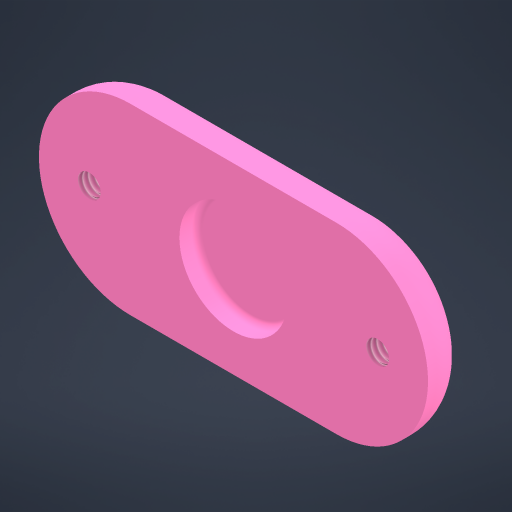
# Autodesk Inventor part: AxleCovers
Saved by Autodesk Inventor 2024.2 (Build 282272000, 272)
## iProperties
Created: 2023-09-28
Part Number: AxleCovers
Material: Generic
Document SubType Name: Modeling
Designer: tech
Density: 1 g/cm^3
Appearance: Machined - Aluminum
Author: tech
Autodesk Inventor part; units mm, degrees
ref_plane "YZ Plane" through (0, 0, 0) normal (1, 0, 0) x (0, 1, 0)
ref_plane "XZ Plane" through (0, 0, 0) normal (0, 1, 0) x (-1, 0, 0)
ref_plane "XY Plane" through (0, 0, 0) normal (0, 0, 1) x (1, 0, 0)
sketch "Sketch10" plane through (0, 0, 0) normal (0, 0, 1) x (1, 0, 0)
  circle A0 centre (0, 0) radius 6
  line L0 (0, 0) -> (16.002, 0)
  line L1 (0, 0) -> (-16.002, 0)
  circle A1 centre (-16.002, 0) radius 1.27
  circle A2 centre (16.002, 0) radius 1.27
  line L2 (-11.43, 10.16) -> (11.43, 10.16)
  line L3 (21.59, 0) -> (21.59, 0)
  line L4 (11.43, -10.16) -> (-11.43, -10.16)
  line L5 (-21.59, 0) -> (-21.59, 0)
  arc A3 (-11.43, 10.16) -> (-21.59, 0) centre (-11.43, 0) ccw
  arc A4 (-21.59, 0) -> (-11.43, -10.16) centre (-11.43, 0) ccw
  arc A5 (11.43, -10.16) -> (21.59, 0) centre (11.43, 0) ccw
  arc A6 (21.59, 0) -> (11.43, 10.16) centre (11.43, 0) ccw
  point P0 (0, -10.16)
  dimension "d40" = 12
  dimension "d41" = 16.002
  dimension "d42" = 16.002
  dimension "d43" = 2.54
  dimension "d44" = 2.54
  dimension "d45" = 10.16
  dimension "d46" = 10.16
  dimension "d47" = 21.59
  dimension "d48" = 21.59
  dimension "d49" = 10.16
  dimension "d50" = 10.16
  dimension "d51" = 10.16
  dimension "d52" = 10.16
  constraints: 12 end point, 8 point on circle, 8 tangent, 7 centre point, 3 coincident, 3 horizontal, 2 parallel, 1 midpoint, 1 perpendicular
  measures "d40" diameter of A0
  measures "d41" distance of L0.start L0.end
  measures "d42" distance of L0.start L1.end
  measures "d43" diameter of A1
  measures "d44" diameter of A2
  measures "d45" distance from line of L2 point (0, 0)
  measures "d46" distance of point (0, -10.16) point (0, 0)
  measures "d47" distance from line of point (0, 0) L3
  measures "d48" distance from line of L5 point (0, 0)
  measures "d49" radius of A3
  measures "d50" radius of A4
  measures "d51" radius of A5
  measures "d52" radius of A6
extrude "Extrusion11" add sketch "Sketch10" against normal blind 5 contours L0 L1 A0 | A1 | A0 L1 L0 | A2 | L2 A6 A5 L4 A4 A3
extrude "Extrusion12" cut sketch "Sketch10" against normal blind 2 contours L0 L1 A0 | A0 L1 L0
fillet "Fillet2" radius 0.635 1 edges at (-6, 0, -2)
fillet "Fillet3" radius 4 4 edges at (0, -10.16, -5) (-21.59, 0, -5) (0, 10.16, -5) (21.59, 0, -5)
extrude "Extrusion13" cut sketch "Sketch10" against normal blind 3.5 contours A1 | A2
thread "Thread1" size "4-40 UNC" class "2B" standard "ANSI Unified Screw Threads" full length
thread "Thread2" size "4-40 UNC" class "2B" standard "ANSI Unified Screw Threads" full length
sketch "Sketch11" plane through (0, 0, -5) normal (0, 0, -1) x (-1, 0, 0)
  line L0 (-21.5717, 10.2034) -> (21.5609, 10.2034) construction
  line L1 (21.5609, 10.2034) -> (21.5609, -10.088) construction
  line L2 (21.5609, -10.088) -> (-21.5717, -10.088) construction
  line L3 (-21.5717, -10.088) -> (-21.5717, 10.2034) construction
  spline S0 degree 2 poles (-8.7726, -2.4036) (-8.7726, -3.0619) (-9.24, -4.0827) (-10.1273, -4.7886) (-11.4247, -5.1511) (-12.2547, -5.1511) knots 0 0 0 1 2 3 4 4 4
  spline S1 degree 2 poles (-12.2547, -5.1511) (-13.0369, -5.1511) (-14.2676, -4.8268) (-15.1357, -4.1781) (-15.5841, -3.2431) (-15.5841, -2.6421) knots 0 0 0 1 2 3 4 4 4
  spline S2 degree 2 poles (-15.5841, -2.6421) (-15.5841, -2.1651) (-15.2693, -1.3638) (-14.6873, -0.696) (-13.8287, -0.1045) (-13.285, 0.1626) knots 0 0 0 1 2 3 4 4 4
  spline S3 degree 2 poles (-13.285, 0.1626) (-13.7524, 0.4011) (-14.4774, 0.9449) (-14.9735, 1.5745) (-15.2311, 2.29) (-15.2311, 2.7193) knots 0 0 0 1 2 3 4 4 4
  spline S4 degree 2 poles (-15.2311, 2.7193) (-15.2311, 3.244) (-14.8495, 4.1789) (-14.0768, 4.8658) (-12.8843, 5.2665) (-12.0829, 5.2665) knots 0 0 0 1 2 3 4 4 4
  spline S5 degree 2 poles (-12.0829, 5.2665) (-11.3197, 5.2665) (-10.2036, 4.8944) (-9.4785, 4.2648) (-9.1351, 3.4062) (-9.1351, 2.9101) knots 0 0 0 1 2 3 4 4 4
  spline S6 degree 2 poles (-9.1351, 2.9101) (-9.1351, 2.5094) (-9.3927, 1.7749) (-9.8888, 1.1261) (-10.6138, 0.5537) (-11.0908, 0.2962) knots 0 0 0 1 2 3 4 4 4
  spline S7 degree 2 poles (-11.0908, 0.2962) (-10.5279, 0.029) (-9.6598, -0.5529) (-9.0779, -1.2207) (-8.7726, -1.9648) (-8.7726, -2.4036) knots 0 0 0 1 2 3 4 4 4
  spline S8 degree 2 poles (-10.1368, -2.5467) (-10.1368, -2.1842) (-10.4039, -1.6023) (-10.9381, -1.0871) (-11.7395, -0.6101) (-12.2737, -0.3525) knots 0 0 0 1 2 3 4 4 4
  spline S9 degree 2 poles (-12.2737, -0.3525) (-12.7603, -0.6006) (-13.5044, -1.0871) (-13.9814, -1.6023) (-14.2199, -2.1747) (-14.2199, -2.5181) knots 0 0 0 1 2 3 4 4 4
  spline S10 degree 2 poles (-14.2199, -2.5181) (-14.2199, -3.2718) (-13.18, -4.1017) (-12.1593, -4.1017) knots 0 0 0 1 2 2 2
  spline S11 degree 2 poles (-12.1593, -4.1017) (-11.1576, -4.1017) (-10.1368, -3.2622) (-10.1368, -2.5467) knots 0 0 0 1 2 2 2
  spline S12 degree 2 poles (-10.4611, 2.7861) (-10.4611, 3.1104) (-10.6901, 3.6447) (-11.1289, 4.0263) (-11.7681, 4.2171) (-12.1879, 4.2171) knots 0 0 0 1 2 3 4 4 4
  spline S13 degree 2 poles (-12.1879, 4.2171) (-13.0274, 4.2171) (-13.8955, 3.4539) (-13.8955, 2.7861) knots 0 0 0 1 2 2 2
  spline S14 degree 2 poles (-13.8955, 2.7861) (-13.8955, 2.4808) (-13.6856, 1.9561) (-13.2373, 1.4887) (-12.5599, 1.0403) (-12.0925, 0.8018) knots 0 0 0 1 2 3 4 4 4
  spline S15 degree 2 poles (-12.0925, 0.8018) (-11.3007, 1.212) (-10.4611, 2.1946) (-10.4611, 2.7861) knots 0 0 0 1 2 2 2
  spline S16 degree 2 poles (-0.4633, -2.127) (-0.4633, -2.3845) (-0.6255, -2.6803) (-0.7591, -2.6803) knots 0 0 0 1 2 2 2
  line L4 (-0.7591, -2.6803) -> (-1.9039, -2.6803)
  line L5 (-1.9039, -2.6803) -> (-1.9039, -4.8077)
  spline S17 degree 2 poles (-1.9039, -4.8077) (-1.9039, -4.8649) (-1.9706, -4.9508) (-2.1328, -5.0176) (-2.3904, -5.0462) (-2.5907, -5.0462) knots 0 0 0 1 2 3 4 4 4
  spline S18 degree 2 poles (-2.5907, -5.0462) (-2.7815, -5.0462) (-3.0391, -5.0176) (-3.1917, -4.9508) (-3.249, -4.8649) (-3.249, -4.8077) knots 0 0 0 1 2 3 4 4 4
  line L6 (-3.249, -4.8077) -> (-3.249, -2.6803)
  line L7 (-3.249, -2.6803) -> (-7.3893, -2.6803)
  spline S19 degree 2 poles (-7.3893, -2.6803) (-7.4752, -2.6803) (-7.5992, -2.6326) (-7.7041, -2.5086) (-7.7423, -2.2701) (-7.7423, -2.0888) knots 0 0 0 1 2 3 4 4 4
  spline S20 degree 2 poles (-7.7423, -2.0888) (-7.7423, -1.9362) (-7.7232, -1.7072) (-7.685, -1.5069) (-7.5992, -1.3352) (-7.5515, -1.2302) knots 0 0 0 1 2 3 4 4 4
  line L8 (-7.5515, -1.2302) -> (-3.9454, 4.923)
  spline S21 degree 2 poles (-3.9454, 4.923) (-3.9072, 4.9803) (-3.7546, 5.0757) (-3.5161, 5.1424) (-3.1631, 5.1615) (-2.9246, 5.1615) knots 0 0 0 1 2 3 4 4 4
  spline S22 degree 2 poles (-2.9246, 5.1615) (-2.6575, 5.1615) (-2.2664, 5.1234) (-2.0279, 5.0566) (-1.9039, 4.9612) (-1.9039, 4.8849) knots 0 0 0 1 2 3 4 4 4
  line L9 (-1.9039, 4.8849) -> (-1.9039, -1.5737)
  line L10 (-1.9039, -1.5737) -> (-0.7591, -1.5737)
  spline S23 degree 2 poles (-0.7591, -1.5737) (-0.6255, -1.5737) (-0.4633, -1.8503) (-0.4633, -2.127) knots 0 0 0 1 2 2 2
  line L11 (-3.249, 3.9786) -> (-3.2681, 3.9786)
  line L12 (-3.2681, 3.9786) -> (-6.5116, -1.5737)
  line L13 (-6.5116, -1.5737) -> (-3.249, -1.5737)
  line L14 (-3.249, -1.5737) -> (-3.249, 3.9786)
  spline S24 degree 2 poles (7.5502, 0.0767) (7.5502, -1.0871) (7.1877, -3.0046) (6.3291, -4.3879) (4.9553, -5.1511) (3.9441, -5.1511) knots 0 0 0 1 2 3 4 4 4
  spline S25 degree 2 poles (3.9441, -5.1511) (2.9997, -5.1511) (1.6927, -4.4738) (0.8913, -3.1477) (0.5574, -1.2207) (0.5574, 0.0386) knots 0 0 0 1 2 3 4 4 4
  spline S26 degree 2 poles (0.5574, 0.0386) (0.5574, 1.1929) (0.9295, 3.12) (1.7786, 4.5033) (3.1523, 5.2665) (4.154, 5.2665) knots 0 0 0 1 2 3 4 4 4
  spline S27 degree 2 poles (4.154, 5.2665) (5.108, 5.2665) (6.4149, 4.5891) (7.2163, 3.2631) (7.5502, 1.336) (7.5502, 0.0767) knots 0 0 0 1 2 3 4 4 4
  spline S28 degree 2 poles (6.1764, -0.0091) (6.1764, 0.7445) (6.0715, 1.9466) (5.8521, 2.8719) (5.5182, 3.5302) (5.0507, 3.969) (4.4497, 4.1598) (4.0777, 4.1598) knots 0 0 0 1 2 3 4 5 6 6 6
  spline S29 degree 2 poles (4.0777, 4.1598) (3.4099, 4.1598) (2.5799, 3.5302) (2.1029, 2.4426) (1.9312, 0.9735) (1.9312, 0.1244) knots 0 0 0 1 2 3 4 4 4
  spline S30 degree 2 poles (1.9312, 0.1244) (1.9312, -1.0013) (2.1697, -2.5944) (2.6753, -3.5866) (3.4671, -4.0445) (4.03, -4.0445) knots 0 0 0 1 2 3 4 4 4
  spline S31 degree 2 poles (4.03, -4.0445) (4.4688, -4.0445) (5.1271, -3.7678) (5.6041, -3.2431) (5.9189, -2.5086) (6.1097, -1.6118) (6.1764, -0.572) (6.1764, -0.0091) knots 0 0 0 1 2 3 4 5 6 6 6
  spline S32 degree 2 poles (15.6591, 0.0767) (15.6591, -1.0871) (15.2966, -3.0046) (14.438, -4.3879) (13.0643, -5.1511) (12.053, -5.1511) knots 0 0 0 1 2 3 4 4 4
  spline S33 degree 2 poles (12.053, -5.1511) (11.1086, -5.1511) (9.8016, -4.4738) (9.0003, -3.1477) (8.6664, -1.2207) (8.6664, 0.0386) knots 0 0 0 1 2 3 4 4 4
  spline S34 degree 2 poles (8.6664, 0.0386) (8.6664, 1.1929) (9.0384, 3.12) (9.8875, 4.5033) (11.2612, 5.2665) (12.2629, 5.2665) knots 0 0 0 1 2 3 4 4 4
  spline S35 degree 2 poles (12.2629, 5.2665) (13.2169, 5.2665) (14.5239, 4.5891) (15.3252, 3.2631) (15.6591, 1.336) (15.6591, 0.0767) knots 0 0 0 1 2 3 4 4 4
  spline S36 degree 2 poles (14.2854, -0.0091) (14.2854, 0.7445) (14.1804, 1.9466) (13.961, 2.8719) (13.6271, 3.5302) (13.1597, 3.969) (12.5586, 4.1598) (12.1866, 4.1598) knots 0 0 0 1 2 3 4 5 6 6 6
  spline S37 degree 2 poles (12.1866, 4.1598) (11.5188, 4.1598) (10.6888, 3.5302) (10.2118, 2.4426) (10.0401, 0.9735) (10.0401, 0.1244) knots 0 0 0 1 2 3 4 4 4
  spline S38 degree 2 poles (10.0401, 0.1244) (10.0401, -1.0013) (10.2786, -2.5944) (10.7842, -3.5866) (11.576, -4.0445) (12.1389, -4.0445) knots 0 0 0 1 2 3 4 4 4
  spline S39 degree 2 poles (12.1389, -4.0445) (12.5777, -4.0445) (13.236, -3.7678) (13.713, -3.2431) (14.0278, -2.5086) (14.2186, -1.6118) (14.2854, -0.572) (14.2854, -0.0091) knots 0 0 0 1 2 3 4 5 6 6 6
  point P0 (0, 0)
  dimension "d40" = 12
  dimension "d41" = 16.002
  dimension "d42" = 16.002
  dimension "d43" = 2.54
  dimension "d44" = 2.54
  constraints: 2 other
extrude "Extrusion14" cut sketch "Sketch11" against normal blind 0.5
body "Solid3"
